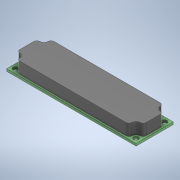
# Autodesk Inventor part: IMU-Measurement-and-Transmission-Module
Saved by Autodesk Inventor 2022 (Build 260153000, 153)
## iProperties
Created: 2023-09-11
Part Number: IMU-Measurement-and-Transmission-Module
Material: 一般
Document SubType Name: Modeling
Designer: Masato Kubotera
Density: 1 g/cm^3
Appearance: 既定
Author: Masato Kubotera
Autodesk Inventor part; units mm, degrees
ref_plane "YZ Plane" through (0, 0, 0) normal (1, 0, 0) x (0, 1, 0)
ref_plane "XZ Plane" through (0, 0, 0) normal (0, 1, 0) x (-1, 0, 0)
ref_plane "XY Plane" through (0, 0, 0) normal (0, 0, 1) x (1, 0, 0)
sketch "スケッチ1" plane through (0, 0, 0) normal (0, 0, 1) x (1, 0, 0)
  line L0 (-12.5, -43.5) -> (12.5, -43.5)
  line L1 (12.5, -43.5) -> (12.5, 43.5)
  line L2 (12.5, 43.5) -> (-12.5, 43.5)
  line L3 (-12.5, 43.5) -> (-12.5, -43.5)
  line L4 (-12.5, -43.5) -> (12.5, 43.5) construction
  line L5 (12.5, -43.5) -> (-12.5, 43.5) construction
  line L6 (9.6, -40.6) -> (-9.6, -40.6) construction
  line L7 (-9.6, -40.6) -> (-9.6, 40.6) construction
  line L8 (-9.6, 40.6) -> (9.6, 40.6) construction
  line L9 (9.6, 40.6) -> (9.6, -40.6) construction
  line L10 (9.6, -40.6) -> (-9.6, 40.6) construction
  line L11 (-9.6, -40.6) -> (9.6, 40.6) construction
  circle A0 centre (-9.6, -40.6) radius 1.6
  circle A1 centre (-9.6, 40.6) radius 1.6
  circle A2 centre (9.6, 40.6) radius 1.6
  circle A3 centre (9.6, -40.6) radius 1.6
  arc A4 (-7.4091, -42.5) -> (-11.5, -38.4091) centre (-9.6, -40.6) ccw
  line L12 (-7.4091, -42.5) -> (7.4091, -42.5)
  line L13 (0, -43.5) -> (0, 43.5) construction
  line L14 (-12.5, 0) -> (12.5, 0) construction
  arc A5 (11.5, -38.4091) -> (7.4091, -42.5) centre (9.6, -40.6) ccw
  arc A6 (-11.5, 38.4091) -> (-7.4091, 42.5) centre (-9.6, 40.6) ccw
  line L15 (-7.4091, 42.5) -> (7.4091, 42.5)
  arc A7 (7.4091, 42.5) -> (11.5, 38.4091) centre (9.6, 40.6) ccw
  line L16 (-11.5, -38.4091) -> (-11.5, 38.4091)
  line L17 (11.5, -38.4091) -> (11.5, 38.4091)
  point P0 (0, 0)
  dimension "d0" = 25
  dimension "d1" = 87
  dimension "d2" = 19.2
  dimension "d3" = 81.2
  dimension "d4" = 3.2
  dimension "d5" = 1
  dimension "d6" = 1
  constraints: 36 end point, 9 symmetric about line, 8 centre point, 8 midpoint, 8 point on circle, 5 coincident, 4 parallel, 3 equal radius, 3 horizontal, 2 perpendicular, 1 tangent, 1 vertical, 3 other
  measures "d0" distance of L2.end L1.end
  measures "d1" distance of L1.end L0.end
  measures "d2" distance of L7.end L8.end
  measures "d3" distance of L8.end L6.start
  measures "d4" diameter of A0
  measures "d5" distance between parallel lines of L16 L3
  measures "d6" distance between parallel lines of L0 L12
extrude "押し出し1" add sketch "スケッチ1" along normal blind 1.6 contours L3 L2 L1 L0 | A4 L16 A6 L15 A7 L17 A5 L12
extrude "押し出し2" add sketch "スケッチ1" along normal blind 9.34 contours A4 L16 A6 L15 A7 L17 A5 L12
fillet "フィレット1" radius 2 8 edges at (11.5, -38.4091, 5.47) (7.4091, -42.5, 5.47) (-7.4091, -42.5, 5.47) (-11.5, -38.4091, 5.47) (11.5, 38.4091, 5.47) (7.4091, 42.5, 5.47) (-7.4091, 42.5, 5.47) (-11.5, 38.4091, 5.47)
equation "\"d6\" = d5"
